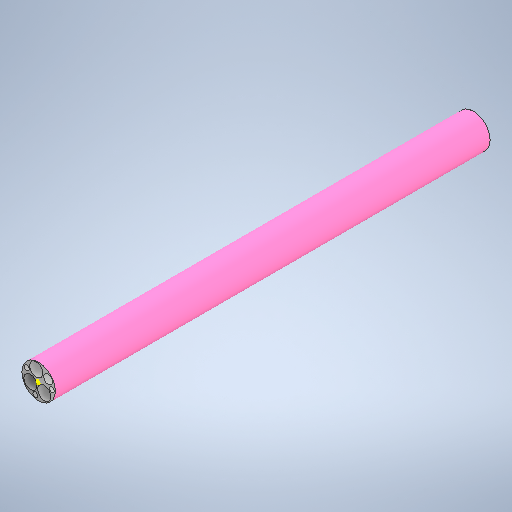
# Autodesk Inventor part: outer casing
Saved by Autodesk Inventor 2025.2 (Build 292293000, 293)
## iProperties
Created: 2025-03-12
Part Number: outer casing
Material: Generic
Document SubType Name: Modeling
Designer: avnr2
Density: 1 g/cm^3
Appearance: Default
Author: avnr2
Autodesk Inventor part; units mm, degrees
ref_plane "YZ Plane" through (0, 0, 0) normal (1, 0, 0) x (0, 1, 0)
ref_plane "XZ Plane" through (0, 0, 0) normal (0, 1, 0) x (-1, 0, 0)
ref_plane "XY Plane" through (0, 0, 0) normal (0, 0, 1) x (1, 0, 0)
sketch "Sketch1" plane through (0, 0, 0) normal (0, 1, 0) x (-1, 0, 0)
  circle A0 centre (0, 0) radius 5
  circle A1 centre (0.7051, 2.7925) radius 2
  circle A2 centre (-1.6909, -2.1323) radius 2
  circle A3 centre (2.4362, -1.3202) radius 2
  circle A4 centre (-2.8575, 2.0067) radius 1.35
  circle A5 centre (3.5172, 1.7971) radius 0.75
  circle A6 centre (0.9671, -3.8612) radius 0.75
  circle A7 centre (-3.984, -0.1323) radius 0.75
  point P0 (2.4362, -7.492)
  point P1 (2.4362, -7.492)
  dimension "d0" = 10
  dimension "d1" = 4
  dimension "d2" = 4
  dimension "d3" = 4
  dimension "d5" = 2.7
  dimension "d6" = 1.5
  dimension "d7" = 1.5
  dimension "d8" = 1.5
  constraints: 8 centre point, 2 coincident
  measures "d0" diameter of A0
  measures "d1" diameter of A1
  measures "d2" diameter of A2
  measures "d3" diameter of A3
  measures "d5" diameter of A4
  measures "d6" diameter of A6
  measures "d7" diameter of A5
  measures "d8" diameter of A7
extrude "Extrusion1" add sketch "Sketch1" along normal blind 130
sketch "Sketch2" plane through (0, 0, 0) normal (0, -1, 0) x (1, 0, 0)
  point P0 (0, 0)
sketch "Sketch3" plane through (0, 0, 0) normal (0, -1, 0) x (1, 0, 0)
  point P0 (0, 0)
body "Solid1"
